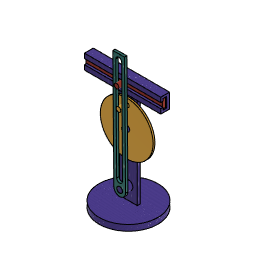
Scotch Yoke Mechanism v3 (Autodesk Fusion 360 design; units mm, degrees)
Autodesk Fusion 360 part; units mm, degrees
note: some values were not read from the file. Set by a fixed rule: which face or edge a step refers to.
sketch "holder-stand" plane through (0, 0, 0) normal (0, 0, 1) x (1, 0, 0)
  circle A0 centre (0, 0) radius 50
  dimension "d2" = 100
  constraint coincident A0.centre origin
  measures "d2" diameter of A0
extrude "Extrude1" add sketch "holder-stand" along normal blind 10 makes body 1
sketch "holder" plane through (0, 0, 10) normal (0, 0, 1) x (-1, 0, 0)
  circle A0 centre (0, 0) radius 50
  line L0 (0, 0) -> (-15, 0)
  line L1 (-15, 0) -> (-15, -5)
  line L2 (-15, -5) -> (0, -5)
  line L3 (0, -5) -> (0, 0)
  line L4 (0, 0) -> (15, 0)
  line L5 (15, -5) -> (0, -5)
  line L6 (15, 0) -> (15, -5)
  dimension "d5" = 15
  dimension "d6" = 5
  constraint horizontal L0
  constraint vertical L1
  constraint horizontal L2
  constraint vertical L3
  constraint coincident A0.centre L0.start
  constraint symmetric A0.centre L3 L0.start
  constraint symmetric L0.end L3 L4.end
  constraint symmetric L1.end L3 L5.start
  constraint symmetric L2.end L3 L5.end
  measures "d5" distance of A0.centre L0.end
  measures "d6" distance of A0.centre L2.end
extrude "Extrude2" cut sketch "holder" against normal blind 35 contours L0 L1 L2 L3 | L3 L4 L5 L6 bodies 1
extrude "Extrude3" add sketch "holder" along normal blind 190 separate body contours L0 L1 L2 L3 | L3 L4 L5 L6 makes body 2
extrude "Extrude4" add 1 faces at (5, 3.3333, 10) along direction (0, 0, -1) blind 10 on bodies 2 bodies 2
sketch "crank-holder" plane through (0, 0, 0) normal (0, -1, 0) x (1, 0, 0)
  line L0 (15, 0) -> (15, 200)
  line L1 (15, 200) -> (-15, 200)
  line L2 (-15, 200) -> (-15, 0)
  line L3 (-15, 0) -> (15, 0)
  line L4 (0, 200) -> (0, 118)
  circle A0 centre (0, 118) radius 5
  dimension "d13" = 82
  dimension "d14" = 10
  constraint midpoint L1 L4.start
  constraint perpendicular L1 L4
  constraint coincident L4.end A0.centre
  measures "d13" distance of L4.start L4.end
  measures "d14" diameter of A0
extrude "Extrude5" add sketch "crank-holder" along normal blind 7 contours A0 bodies 2
sketch "crank" plane through (0, 0, 0) normal (0, -1, 0) x (1, 0, 0)
  circle A0 centre (0, 118) radius 5
  line L0 (15, 0) -> (15, 200)
  line L1 (15, 200) -> (-15, 200)
  line L2 (-15, 200) -> (-15, 0)
  line L3 (-15, 0) -> (15, 0)
  circle A1 centre (0, 118) radius 45
  dimension "d17" = 90
  constraint concentric A0 A1
  measures "d17" diameter of A1
extrude "Extrude6" add sketch "crank" along normal blind 3 separate body contours A0 | L0 L2 A1 | L0 A1 | L2 A1 makes body 3
extrude "Extrude7" cut sketch "crank-holder" along normal blind 10 contours A0 bodies 3
move_face "OffsetFaces1" offset -0.3 1 faces at (-4.6074, -2.3333, 119.9422) on bodies 2
sketch "slider-holder-right" plane through (15, 0, 0) normal (1, 0, 0) x (0, 1, 0)
  line L0 (5, 0) -> (5, 200)
  line L1 (5, 200) -> (0, 200)
  line L2 (0, 200) -> (0, 0)
  line L3 (0, 0) -> (5, 0)
  line L4 (0, 200) -> (5, 200)
  line L5 (5, 200) -> (5, 175)
  line L6 (5, 175) -> (0, 175)
  line L7 (0, 175) -> (0, 200)
  dimension "d23" = 25
  constraint horizontal L4
  constraint vertical L5
  constraint horizontal L6
  constraint vertical L7
  constraint coincident L1.end L2.start
  measures "d23" distance of L1.end L6.end
sketch "slider-holder-left" plane through (-15, 0, 0) normal (-1, 0, 0) x (0, -1, 0)
  line L0 (0, 0) -> (0, 200)
  line L1 (0, 200) -> (-5, 200)
  line L2 (-5, 200) -> (-5, 0)
  line L3 (-5, 0) -> (0, 0)
  line L4 (-5, 200) -> (0, 200)
  line L5 (0, 200) -> (0, 175)
  line L6 (0, 175) -> (-5, 175)
  line L7 (-5, 175) -> (-5, 200)
  dimension "d24" = 25
  constraint horizontal L4
  constraint vertical L5
  constraint horizontal L6
  constraint vertical L7
  constraint coincident L1.end L2.start
  measures "d24" distance of L1.end L6.end
extrude "Extrude8" add sketch "slider-holder-right" along normal blind 50 contours L0 L1 L2 L4 L5 L6 L7 bodies 2
extrude "Extrude9" add sketch "slider-holder-left" along normal blind 50 contours L0 L1 L2 L4 L5 L6 L7 bodies 2
sketch "slider-holder-front" plane through (0, 0, 0) normal (0, -1, 0) x (1, 0, 0)
  circle A0 centre (0, 118) radius 4.7
  line L0 (15, 0) -> (15, 175)
  line L1 (15, 175) -> (65, 175)
  line L2 (65, 175) -> (65, 200)
  line L3 (65, 200) -> (-65, 200)
  line L4 (-65, 200) -> (-65, 175)
  line L5 (-65, 175) -> (-15, 175)
  line L6 (-15, 175) -> (-15, 0)
  line L7 (-15, 0) -> (15, 0)
  line L8 (-65, 200) -> (65, 200)
  line L9 (65, 200) -> (65, 196)
  line L10 (65, 196) -> (-65, 196)
  line L11 (-65, 196) -> (-65, 200)
  line L12 (-65, 175) -> (65, 175)
  line L13 (65, 175) -> (65, 179)
  line L14 (65, 179) -> (-65, 179)
  line L15 (-65, 179) -> (-65, 175)
  dimension "d29" = 4
  dimension "d30" = 4
  constraint horizontal L8
  constraint vertical L9
  constraint horizontal L10
  constraint vertical L11
  constraint coincident L2 L9.end
  constraint coincident L3.end L4.start
  constraint horizontal L12
  constraint vertical L13
  constraint horizontal L14
  constraint vertical L15
  constraint coincident L2 L13.end
  constraint coincident L4.end L5.start
  measures "d29" distance of L3.end L10.end
  measures "d30" distance of L4.end L14.end
extrude "Extrude10" add sketch "slider-holder-front" along normal blind 10 contours L1 L2 L4 L5 L12 L13 L14 L15 | L2 L3 L4 L8 L9 L10 L11 bodies 2
sketch "slider-barrier-bottom" plane through (0, 0, 179) normal (0, 0, 1) x (-1, 0, 0)
  line L0 (-65, 0) -> (65, 0)
  line L1 (65, 0) -> (65, 10)
  line L2 (65, 10) -> (-65, 10)
  line L3 (-65, 10) -> (-65, 0)
  line L4 (65, 10) -> (-65, 10)
  line L5 (-65, 10) -> (-65, 6)
  line L6 (-65, 6) -> (65, 6)
  line L7 (65, 6) -> (65, 10)
  dimension "d33" = 4
  constraint horizontal L4
  constraint vertical L5
  constraint horizontal L6
  constraint vertical L7
  constraint coincident L3 L5.end
  constraint coincident L1.end L2.start
  measures "d33" distance of L1.end L6.end
sketch "slider-barrier-top" plane through (0, 0, 196) normal (0, 0, -1) x (1, 0, 0)
  line L0 (-65, 0) -> (65, 0)
  line L1 (65, 0) -> (65, 10)
  line L2 (65, 10) -> (-65, 10)
  line L3 (-65, 10) -> (-65, 0)
  line L4 (-65, 10) -> (65, 10)
  line L5 (65, 10) -> (65, 6)
  line L6 (65, 6) -> (-65, 6)
  line L7 (-65, 6) -> (-65, 10)
  dimension "d34" = 4
  constraint horizontal L4
  constraint vertical L5
  constraint horizontal L6
  constraint vertical L7
  constraint coincident L1 L5.end
  constraint coincident L2.end L3.start
  measures "d34" distance of L2.end L6.end
extrude "Extrude11" add sketch "slider-barrier-top" along normal blind 4 contours L1 L2 L3 L4 L5 L6 L7 bodies 2
extrude "Extrude12" add sketch "slider-barrier-bottom" along normal blind 4 contours L1 L2 L3 L4 L5 L6 L7 bodies 2
sketch "slider" plane through (65, 0, 0) normal (1, 0, 0) x (0, 1, 0)
  line L0 (-10, 175) -> (5, 175)
  line L1 (5, 175) -> (5, 200)
  line L2 (5, 200) -> (-10, 200)
  line L3 (-10, 200) -> (-10, 192)
  line L4 (-10, 192) -> (-6, 192)
  line L5 (-6, 192) -> (-6, 196)
  line L6 (-6, 196) -> (0, 196)
  line L7 (0, 196) -> (0, 179)
  line L8 (0, 179) -> (-6, 179)
  line L9 (-6, 179) -> (-6, 183)
  line L10 (-6, 183) -> (-10, 183)
  line L11 (-10, 183) -> (-10, 175)
  line L12 (-6, 196) -> (0, 196)
  line L13 (0, 196) -> (0, 179)
  line L14 (0, 179) -> (-6, 179)
  line L15 (-6, 179) -> (-6, 196)
  constraint horizontal L12
  constraint vertical L13
  constraint horizontal L14
  constraint vertical L15
  constraint coincident L7.end L8.start
  constraint coincident L5.end L6.start
extrude "Extrude13" add sketch "slider" against normal blind 130 separate body contours L5 L6 L7 L8 L9 L12 L13 L14 L15 makes body 4
move_face "OffsetFaces2" offset -0.3 6 faces at (21.6667, -4, 196) (21.6667, -6, 186) (-21.6667, -6, 193.3333) (-21.6667, -6, 180.3333) (-21.6667, 0, 190.3333) (21.6667, -2, 179) on bodies 4
sketch "link-holder" plane through (0, 0, 0) normal (0, -1, 0) x (1, 0, 0)
  line L0 (15, 175) -> (-15, 175)
  line L1 (-15, 175) -> (-15, 0)
  line L2 (-15, 0) -> (15, 0)
  line L3 (15, 0) -> (15, 175)
  circle A0 centre (0, 118) radius 4.7
  circle A1 centre (0, 33.2281) radius 5
  dimension "d42" = 10
  measures "d42" diameter of A1
extrude "Extrude14" add sketch "link-holder" along normal blind 15 contours A1 bodies 2
sketch "slotted-link" plane through (0, -15, 0) normal (0, -1, 0) x (1, 0, 0)
  circle A0 centre (0, 33.2281) radius 5
  circle A1 centre (0, 33.2281) radius 10
  line L0 (10, 33.2281) -> (-10, 33.2281)
  line L1 (-10, 33.2281) -> (10, 33.2281)
  line L2 (10, 33.2281) -> (10, 233.2281)
  line L3 (10, 233.2281) -> (-10, 233.2281)
  line L4 (-10, 233.2281) -> (-10, 33.2281)
  line L5 (-5, 33.2281) -> (5, 33.2281)
  line L6 (5, 33.2281) -> (5, 228.2281)
  line L7 (5, 228.2281) -> (-5, 228.2281)
  line L8 (-5, 228.2281) -> (-5, 33.2281)
  circle A2 centre (0, 48.2281) radius 5
  circle A3 centre (0, 223.2281) radius 5
  dimension "d45" = 5
  dimension "d46" = 20
  dimension "d47" = 200
  dimension "d48" = 10
  dimension "d49" = 195
  dimension "d50" = 10
  constraint coincident A1 L0.start
  constraint coincident A1 L0.end
  constraint horizontal L0
  constraint horizontal L1
  constraint vertical L2
  constraint horizontal L3
  constraint vertical L4
  constraint horizontal L5
  constraint vertical L6
  constraint horizontal L7
  constraint vertical L8
  constraint coincident L1 L5.start
  constraint coincident A0 L5.start
  constraint tangent L6 A2
  constraint tangent L8 A2
  constraint tangent A1 A2
  constraint tangent L7 A3
  measures "d45" distance of A0
  measures "d46" distance of L0.end L0.start
  measures "d47" distance of L0.end L3.end
  measures "d48" distance of L5.start L5.end
  measures "d49" distance of L5.start L7.end
  measures "d50" diameter of A3
extrude "Extrude15" add sketch "slotted-link" against normal blind 4 separate body contours A0 A1 L0 L1 | A1 L0 L1 L6 | A0 A1 L6 L8 | A1 L0 L1 L8 | A1 L2 L3 L4 L6 L7 L8 | A1 L6 A2 | A1 L8 A2 | L6 L7 A3 | L7 L8 A3 makes body 5
move_face "OffsetFaces3" offset -0.3 1 faces at (4.9752, -10, 32.7303) on bodies 2
sketch "slotted-link-holder" plane through (0, -15, 0) normal (0, -1, 0) x (1, 0, 0)
  circle A0 centre (0, 33.2281) radius 4.7
  circle A1 centre (0, 33.2281) radius 7.5
  dimension "d54" = 15
  constraint concentric A0 A1
  measures "d54" diameter of A1
extrude "Extrude16" add sketch "slotted-link-holder" along normal blind -15 and the other way blind 4 bodies 2
sketch "crank-pin" plane through (0, -3, 0) normal (0, -1, 0) x (1, 0, 0)
  circle A0 centre (0, 118) radius 5
  circle A1 centre (0, 118) radius 45
  circle A2 centre (0, 83.063) radius 4
  dimension "d59" = 8
  measures "d59" diameter of A2
sketch "slider-pin" plane through (0, -5.7, 0) normal (0, -1, 0) x (1, 0, 0)
  line L0 (65, 179.3) -> (65, 195.7)
  line L1 (65, 195.7) -> (-65, 195.7)
  line L2 (-65, 195.7) -> (-65, 179.3)
  line L3 (-65, 179.3) -> (65, 179.3)
  circle A0 centre (0, 187.345) radius 4
  dimension "d60" = 8
  measures "d60" diameter of A0
extrude "Extrude17" add sketch "slider-pin" along normal blind 13 contours A0 bodies 4
extrude "Extrude18" add sketch "crank-pin" along normal blind 14 contours A2 bodies 3
copy_body "Body->Comp1" bodies 1 removing the originals makes body 6 in component "holder-stand"
copy_body "Body->Comp2" bodies 2 removing the originals makes body 7 in component "holder"
copy_body "Body->Comp3" bodies 3 removing the originals makes body 8 in component "crank"
copy_body "Body->Comp4" bodies 4 removing the originals makes body 9 in component "slider"
copy_body "Body->Comp5" bodies 5 removing the originals makes body 10 in component "slotted-link"
component "holder-stand" placed x (1, 0, 0) y (0, 1, 0) z (0, 0, 1) at (0, 0, 0)
component "holder" placed x (1, 0, 0) y (0, 1, 0) z (0, 0, 1) at (0, 0, 0)
component "crank" placed x (1, 0, 0) y (0, 1, 0) z (0, 0, 1) at (0, 0, 0)
component "slider" placed x (1, 0, 0) y (0, 1, 0) z (0, 0, 1) at (0, 0, 0)
component "slotted-link" placed x (1, 0, 0) y (0, 1, 0) z (0, 0, 1) at (0, 0, 0)
named bodies: "holder-stand", "holder", "crank", "slider", "slotted-link"
